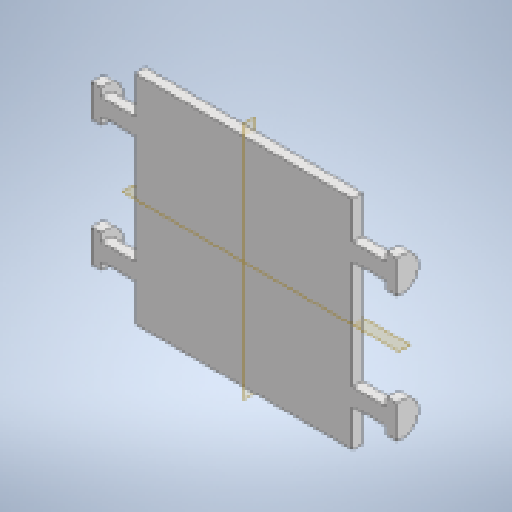
# Autodesk Inventor part: Parte deslizante
Saved by Autodesk Inventor 2024 (Build 280153000, 153)
## iProperties
Created: 2025-03-02
Part Number: Parte deslizante
Material: Genérico
Document SubType Name: Modeling
Designer: sergi
Density: 1 g/cm^3
Appearance: Valor por defecto
Author: sergi
Autodesk Inventor part; units mm, degrees
ref_plane "YZ Plane" through (0, 0, 0) normal (1, 0, 0) x (0, 1, 0)
ref_plane "XZ Plane" through (0, 0, 0) normal (0, 1, 0) x (-1, 0, 0)
ref_plane "XY Plane" through (0, 0, 0) normal (0, 0, 1) x (1, 0, 0)
sketch "Boceto1" plane through (0, 0, 0) normal (0, 0, 1) x (1, 0, 0)
  line L0 (-32, -32) -> (32, -32)
  line L1 (32, -32) -> (32, 32)
  line L2 (32, 32) -> (-32, 32)
  line L3 (-32, 32) -> (-32, -32)
  line L4 (-32, -32) -> (32, 32) construction
  line L5 (32, -32) -> (-32, 32) construction
  point P0 (0, 0)
  dimension "d0" = 64
  dimension "d1" = 64
  constraints: 12 end point, 2 midpoint, 2 parallel, 1 horizontal, 1 perpendicular
  measures "d0" distance of L2.end L1.end
  measures "d1" distance of L1.end L0.end
extrude "Extrusión1" add sketch "Boceto1" along normal blind 3
sketch "Boceto2" plane through (32, -32, 0) normal (1, 0, 0) x (0, 0, -1)
  line L0 (-74, 16.5) -> (1, 16.5) projected
  arc A0 (1, 10.5) -> (1, 16.5) centre (1, 13.5) ccw projected
  line L1 (1, 10.5) -> (-74, 10.5) projected
  line L2 (-74, -4.5) -> (-74, 10.5) projected
  line L3 (7, -4.5) -> (-74, -4.5) projected
  line L4 (7, -4.5) -> (7, 68.5) projected
  line L5 (7, 68.5) -> (-74, 68.5) projected
  line L6 (-74, 53.5) -> (-74, 68.5) projected
  line L7 (-74, 53.5) -> (1, 53.5) projected
  arc A1 (1, 47.5) -> (1, 53.5) centre (1, 50.5) ccw projected
  line L8 (1, 47.5) -> (-74, 47.5) projected
  line L9 (-74, 16.5) -> (-74, 47.5) projected
  line L10 (0, 0) -> (0, 64) projected
  line L11 (0, 64) -> (-3, 64) projected
  line L12 (-3, 0) -> (-3, 64) projected
  line L13 (0, 0) -> (-3, 0) projected
  line L14 (0, 47.5) -> (-3, 47.5)
  line L15 (-3, 47.5) -> (-3, 53.5)
  line L16 (-3, 53.5) -> (0, 53.5)
  line L17 (0, 53.5) -> (0, 47.5)
  line L18 (0, 47.7) -> (-3, 47.7)
  line L19 (-2.8, 47.7) -> (-2.8, 53.3)
  line L20 (-3, 53.3) -> (0, 53.3)
  line L21 (-0.2, 53.3) -> (-0.2, 47.7)
  line L22 (-2.5, 53) -> (-2.5, 48)
  line L23 (-3, 48) -> (0, 48)
  line L24 (-0.5, 48) -> (-0.5, 53)
  line L25 (0, 53) -> (-3, 53)
  point P0 (0, 32)
  dimension "d4" = 0.2
  dimension "d10" = 0.5
  constraints: 24 end point, 20 point on line, 6 parallel, 3 perpendicular, 1 horizontal
  measures "d4" distance between parallel lines of L17 L21
  measures "d10" distance between parallel lines of L15 L22
extrude "Extrusión2" add sketch "Boceto2" along normal blind 10 contours L12 L25 L19 L23 | L23 L21 L25 L10 | L19 L25 L22 L23 | L23 L24 L25 L21 | L22 L25 L24 L23
sketch "Boceto3" plane through (42, -32, 0) normal (1, 0, 0) x (0, 0, -1)
  line L0 (-3, 53) -> (-3, 48) projected
  line L1 (0, 48) -> (0, 53) projected
  line L2 (0, 47.7) -> (-3, 53.3)
  circle A0 centre (-1.5, 50.5) radius 5
  line L3 (-3, 53.3) -> (-3, 55.2697)
  line L4 (-3, 47.7) -> (0, 47.7)
  line L5 (0, 47.7) -> (0, 53.3)
  line L6 (0, 53.3) -> (-3, 53.3)
  line L7 (-3, 53.3) -> (-3, 47.7)
  line L8 (-3, 47.7) -> (-3, 42)
  line L9 (-3, 48) -> (0, 48) projected
  line L10 (0, 53) -> (-3, 53) projected
  point P0 (0, 32)
  point P1 (-3, 45.7303)
  point P2 (-2.8393, 53)
  point P3 (-0.1607, 48)
  dimension "d7" = 10
  constraints: 14 end point, 2 parallel, 1 horizontal, 1 midpoint, 1 perpendicular, 1 vertical, 3 other
extrude "Extrusión3" add sketch "Boceto3" along normal blind 3 contours L10 L2 L9 L0 | L7 L2 L10 | L9 L2 L4 L7 | L6 L5 L10 L2 | L3 A0 L8 L4 L5 L1 L6 | L10 L1 L9 L2 | L9 L5 L2
ref_plane "Plano de trabajo1" through (0, -32, 3) normal (1, 0, 0) x (0, 0, -1)
ref_plane "Plano de trabajo2" through (-32, 0, 0) normal (0, 1, 0) x (1, 0, 0)
mirror "Simetría1" about plane through (-32, 0, 0) normal (0, 1, 0) of "Extrusión2", "Extrusión3"
mirror "Simetría2" about plane through (0, -32, 3) normal (1, 0, 0) of "Extrusión2", "Simetría1", "Extrusión3"
sketch "Boceto4" plane through (0, 0, 3) normal (0, 0, 1) x (1, 0, 0)
  arc A0 (-26.7524, -33.5) -> (-33.5, -26.7524) centre (-31.4, -31.4) ccw projected
  arc A1 (33.5, -26.7524) -> (26.7524, -33.5) centre (31.4, -31.4) ccw projected
  arc A2 (26.7524, 33.5) -> (33.5, 26.7524) centre (31.4, 31.4) ccw projected
  arc A3 (-33.5, 26.7524) -> (-26.7524, 33.5) centre (-31.4, 31.4) ccw projected
  line L0 (32, -32) -> (32, -21) projected
  line L1 (32, -21) -> (42, -21) projected
  line L2 (42, -23.2697) -> (42, -21) projected
  line L3 (42, -23.2697) -> (45, -23.2697) projected
  line L4 (45, -23.2697) -> (45, -13.7303) projected
  line L5 (42, -13.7303) -> (45, -13.7303) projected
  line L6 (42, -16) -> (42, -13.7303) projected
  line L7 (32, -16) -> (42, -16) projected
  line L8 (32, -16) -> (32, 16) projected
  line L9 (32, 16) -> (42, 16) projected
  line L10 (42, 16) -> (42, 13.7303) projected
  line L11 (42, 13.7303) -> (45, 13.7303) projected
  line L12 (45, 23.2697) -> (45, 13.7303) projected
  line L13 (42, 23.2697) -> (45, 23.2697) projected
  line L14 (42, 23.2697) -> (42, 21) projected
  line L15 (32, 21) -> (42, 21) projected
  line L16 (32, 21) -> (32, 32) projected
  line L17 (32, 32) -> (-32, 32) projected
  line L18 (-32, 32) -> (-32, 21) projected
  line L19 (-32, 21) -> (-42, 21) projected
  line L20 (-42, 23.2697) -> (-42, 21) projected
  line L21 (-42, 23.2697) -> (-45, 23.2697) projected
  line L22 (-45, 23.2697) -> (-45, 13.7303) projected
  line L23 (-42, 13.7303) -> (-45, 13.7303) projected
  line L24 (-42, 16) -> (-42, 13.7303) projected
  line L25 (-32, 16) -> (-42, 16) projected
  line L26 (-32, 16) -> (-32, -16) projected
  line L27 (-32, -16) -> (-42, -16) projected
  line L28 (-42, -16) -> (-42, -13.7303) projected
  line L29 (-42, -13.7303) -> (-45, -13.7303) projected
  line L30 (-45, -23.2697) -> (-45, -13.7303) projected
  line L31 (-42, -23.2697) -> (-45, -23.2697) projected
  line L32 (-42, -23.2697) -> (-42, -21) projected
  line L33 (-32, -21) -> (-42, -21) projected
  line L34 (-32, -21) -> (-32, -32) projected
  line L35 (-32, -32) -> (32, -32) projected
  arc A4 (-24.9298, -34.3235) -> (-34.3235, -24.9298) centre (-31.4, -31.4) ccw
  arc A5 (-34.3235, 24.9298) -> (-24.9298, 34.3235) centre (-31.4, 31.4) ccw
  arc A6 (24.9298, 34.3235) -> (34.3235, 24.9298) centre (31.4, 31.4) ccw
  arc A7 (34.3235, -24.9298) -> (24.9298, -34.3235) centre (31.4, -31.4) ccw
  point P0 (0, 0)
  point P1 (-32, 24.3254)
  point P2 (-24.3254, 32)
  point P3 (-24.3254, -32)
  point P4 (-32, -24.3254)
  point P5 (32, -24.3254)
  point P6 (24.3254, -32)
  point P7 (24.3254, 32)
  point P8 (32, 24.3254)
  dimension "d11" = 2
  dimension "d12" = 2
  dimension "d13" = 2
  dimension "d14" = 2
  constraints: 8 point on circle, 4 centre point
  measures "d11" radial gap between concentric circles of A0 A4
  measures "d12" radial gap between concentric circles of A3 A5
  measures "d13" radial gap between concentric circles of A2 A6
  measures "d14" radial gap between concentric circles of A1 A7
extrude "Extrusión4" cut sketch "Boceto4" against normal blind 3 contours L35 L34 A0 | A0 L34 A4 L35 | A7 L0 A1 L35 | A1 L0 L35 | L18 A3 L17 A5 | L18 L17 A3 | A6 L17 A2 L16 | A2 L17 L16
